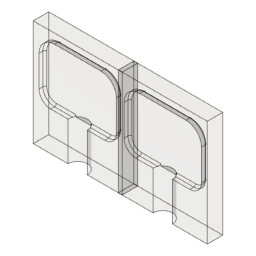
Stillidót v9 (Autodesk Fusion 360 design; units mm, degrees)
Autodesk Fusion 360 part; units mm, degrees
note: some values were not read from the file. Chosen so that the rebuilt part matches the saved one: which bodies a step acts on.
sketch "Sketch1" plane through (0, 0, 0) normal (0, 0, 1) x (1, 0, 0)
  circle A0 centre (25, 25) radius 5
  dimension "d1" = 10
  measures "d1" diameter of A0
extrude "Extrude1" add sketch "Sketch1" along normal blind 20 makes body 1
sketch "Sketch2" plane through (0, 0, 20) normal (0, 0, 1) x (-1, 0, 0)
  circle A0 centre (-25, -25) radius 5
  line L0 (-5, -28) -> (-45, -28)
  line L1 (-45, -28) -> (-45, -22)
  line L2 (-45, -22) -> (-5, -22)
  line L3 (-5, -22) -> (-5, -28)
  constraint horizontal L0
  constraint vertical L1
  constraint horizontal L2
  constraint vertical L3
extrude "Extrude2" add sketch "Sketch2" along normal blind 30 contours A0 L0 L2 | A0 L0 L2 L3 | A0 L0 L1 L2 bodies 1
sketch "Sketch3" plane through (0, 22, 0) normal (0, -1, 0) x (1, 0, 0)
  line L0 (29, 20) -> (45, 20)
  line L1 (45, 20) -> (45, 50)
  line L2 (45, 50) -> (5, 50)
  line L3 (5, 50) -> (5, 20)
  line L4 (5, 20) -> (21, 20)
  line L5 (21, 20) -> (29, 20)
  line L6 (5, 20) -> (20, 20)
  circle A0 centre (10, 25) radius 5
  circle A1 centre (10, 45) radius 5
  circle A2 centre (40, 45) radius 5
  circle A3 centre (40, 25) radius 5
  constraint coincident L3.end L4.start
  constraint coincident L4 L6.end
  constraint perpendicular L3 L6
  constraint tangent L3 A0
  constraint tangent L2 A1
  constraint tangent L2 A2
  constraint tangent L0 A3
fillet "Fillet1" radius 8 1 edges at (5, 25, 50) on bodies 1
fillet "Fillet2" radius 8 1 edges at (45, 25, 50) on bodies 1
fillet "Fillet3" radius 6 1 edges at (5, 25, 20) on bodies 1
fillet "Fillet4" radius 6 1 edges at (45, 25, 20) on bodies 1
fillet "Fillet5" radius 1 9 edges at (16, 22, 20) (6.7574, 22, 21.7574) (5, 22, 34) (7.3431, 22, 47.6569) (25, 22, 50) (42.6569, 22, 47.6569) (45, 22, 34) (43.2426, 22, 21.7574) (34, 22, 20) on bodies 1
fillet "Fillet6" radius 1 9 edges at (34, 28, 20) (43.2426, 28, 21.7574) (45, 28, 34) (42.6569, 28, 47.6569) (25, 28, 50) (7.3431, 28, 47.6569) (5, 28, 34) (6.7574, 28, 21.7574) (16, 28, 20) on bodies 1
sketch "Sketch5" plane through (0, 0, 0) normal (0, 0, 1) x (1, 0, 0)
  line L0 (2, 17) -> (48, 17)
  line L1 (48, 17) -> (48, 33)
  line L2 (48, 33) -> (2, 33)
  line L3 (2, 33) -> (2, 17)
  line L4 (2, 17) -> (48, 33) construction
  line L5 (48, 17) -> (2, 33) construction
  point P0 (25, 25)
  constraint horizontal L0
  constraint perpendicular L0 L1
  constraint parallel L0 L2
  constraint parallel L1 L3
  constraint coincident L4 P0
  constraint coincident L5 P0
extrude "Extrude4" add sketch "Sketch5" along normal blind 55 and the other way blind 0 separate body makes body 2
sketch "Sketch6" plane through (2, 0, 0) normal (-1, 0, 0) x (0, -1, 0)
  line L0 (-17, 0) -> (-17, 55)
  line L1 (-17, 55) -> (-33, 55)
  line L2 (-33, 55) -> (-33, 0)
  line L3 (-33, 0) -> (-17, 0)
  line L4 (-25, 55) -> (-25, 0)
  constraint midpoint L1 L4.start
  constraint midpoint L3 L4.end
sketch "Sketch7" plane through (2, 0, 0) normal (-1, 0, 0) x (0, -1, 0)
  line L0 (-17, 0) -> (-17, 55)
  line L1 (-17, 55) -> (-33, 55)
  line L2 (-33, 55) -> (-33, 0)
  line L3 (-33, 0) -> (-17, 0)
  line L4 (-25, 55) -> (-25, 0)
  constraint midpoint L1 L4.start
  constraint midpoint L3 L4.end
split "Split2" by curves path "Sketch7" along L4 bodies 2 makes body 3 at (32.6667, 33, 18.3333)
combine "Combine1" operation cut target body 2 tool bodies 1 keep tools result as body 4 in component "Component''"
combine "Combine1'" operation cut target body 3 tool bodies 1 keep tools result as body 5 in component "Component'''"
move_body "Move1" bodies 4 to x (1, 0, 0) y (0, 1, 0) z (0, 0, 1) at (-80, 0, 0) in component "Component''"
move_body "Move2" bodies 4 to x (-1, 0, 0) y (0, -1, 0) z (0, 0, 1) at (-64, 50, 0) in component "Component''"
move_body "Move3" bodies 4 to x (1, 0, 0) y (0, 1, 0) z (0, 0, 1) at (-15, 0, 0) in component "Component''"
move_body "Move1'" bodies 5 to x (1, 0, 0) y (0, 1, 0) z (0, 0, 1) at (-5, 0, 0) in component "Component'''"
sketch "Sketch8" plane through (0, 33, 0) normal (0, 1, 0) x (-1, 0, 0)
  line L0 (1, 0) -> (47, 0)
  line L1 (47, 0) -> (47, 55)
  line L2 (47, 55) -> (1, 55)
  line L3 (1, 55) -> (1, 0)
  line L4 (-53, 55) -> (-53, 65)
  line L5 (-53, 65) -> (-43, 65)
  line L6 (57, 0) -> (57, -10)
  line L7 (57, -10) -> (47, -10)
  line L8 (-53, 65) -> (57, 65)
  line L9 (57, 65) -> (57, -10)
  line L10 (57, -10) -> (-53, -10)
  line L11 (-53, -10) -> (-53, 65)
  dimension "d27" = 10
  dimension "d28" = 10
  constraint vertical L4
  constraint horizontal L5
  constraint vertical L6
  constraint horizontal L7
  constraint horizontal L8
  constraint vertical L9
  constraint horizontal L10
  constraint vertical L11
  measures "d27" distance of L0.end L6.start
  measures "d28" distance of L0.end L7.end
extrude "Extrude5" add sketch "Sketch8" against normal blind 30 separate body contours L0 L1 L2 L3 | L4 L5 L6 L7 L8 L9 L10 L11 makes body 6
component "Component'" placed x (1, 0, 0) y (0, 1, 0) z (0, 0, 1) at (0, 0, 0)
component "Component''" placed x (1, 0, 0) y (0, 1, 0) z (0, 0, 1) at (0, 0, 0)
component "Component'''" placed x (1, 0, 0) y (0, 1, 0) z (0, 0, 1) at (0, 0, 0)
hidden bodies 2 3 6
named bodies: "Stock"
